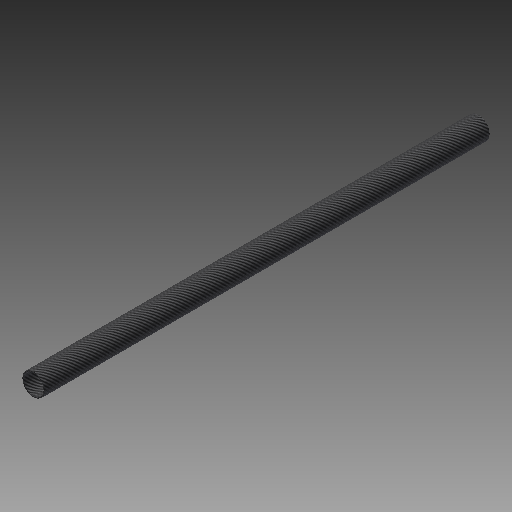
# Autodesk Inventor part: 500mm tube
Saved by Autodesk Inventor 2018 (Build 220112000, 112)
## iProperties
Created: 2018-07-21
Part Number: 500mm tube
Material: CFRP
Document SubType Name: Modeling
Designer: Michael Gunderman
Density: 1.43 g/cm^3
Appearance: Carbon Fiber
Author: Michael Gunderman
Autodesk Inventor part; units mm, degrees
ref_plane "YZ Plane" through (0, 0, 0) normal (1, 0, 0) x (0, 1, 0)
ref_plane "XZ Plane" through (0, 0, 0) normal (0, 1, 0) x (-1, 0, 0)
ref_plane "XY Plane" through (0, 0, 0) normal (0, 0, 1) x (1, 0, 0)
sketch "Sketch1" plane through (0, 0, 0) normal (0, 0, 1) x (1, 0, 0)
  circle A0 centre (0, 0) radius 12.5
  circle A1 centre (0, 0) radius 11.5
  dimension "d0" = 12.5
  dimension "d1" = 11.5
  constraints: 2 centre point, 2 coincident
  measures "d0" radius of A0
  measures "d1" radius of A1
extrude "Extrusion1" add sketch "Sketch1" along normal blind 500
body "Solid1"
